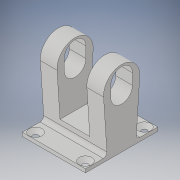
# Autodesk Inventor part: BT101_trajan20_21
Saved by Autodesk Inventor 2022.2 (Build 262287000, 287)
## iProperties
Company: HTBLA Kaindorf
RuleStatus: InUse
Created: 2022-08-03
Part Number: BT101_trajan20_21
Project: Zeichenmaschine_v2
Material: Generisch
Description: halterung
Document SubType Name: Modeling
Designer: trajan20
Density: 1 g/cm^3
Appearance: Vorgabe
Mass: 13.5366 g
Surface Area: 74.1019 cm^2
Volume: 13.5366 cm^3
AfterDocNew0: iProperties-Editor_aufrufen
Author: jan
Keywords: 2021
Autodesk Inventor part; units mm, degrees
ref_plane "YZ Plane" through (0, 0, 0) normal (1, 0, 0) x (0, 1, 0)
ref_plane "XZ Plane" through (0, 0, 0) normal (0, 1, 0) x (-1, 0, 0)
ref_plane "XY Plane" through (0, 0, 0) normal (0, 0, 1) x (1, 0, 0)
sketch "Skizze3" plane through (0, 0, 0) normal (0, 0, 1) x (1, 0, 0)
  line L0 (0, 0) -> (-40, 0)
  line L1 (-40, 0) -> (-40, 35)
  line L2 (-40, 35) -> (0, 35)
  line L3 (0, 35) -> (0, 0)
  point P0 (-3.7, 3.7)
  dimension "d4" = 35
  dimension "d5" = 40
  dimension "d6" = 3.7
  dimension "d7" = 3.7
  constraints: 8 end point, 2 parallel, 1 horizontal, 1 perpendicular
  measures "d4" distance between parallel lines of L2 L0
  measures "d5" distance between parallel lines of L1 L3
  measures "d6" distance from line of L3 point (-3.7, 3.7)
  measures "d7" distance from line of L0 point (-3.7, 3.7)
sketch "Skizze4" plane through (0, 0, 0) normal (0, 1, 0) x (-1, 0, 0)
  line L0 (0, 0) -> (40, 0) projected
  line L1 (20, 0) -> (20, 40)
  line L2 (20, 33) -> (20, 27) construction
  line L3 (26, 33) -> (26, 27)
  line L4 (14, 27) -> (14, 33)
  arc A0 (26, 33) -> (14, 33) centre (20, 33) ccw
  arc A1 (14, 27) -> (26, 27) centre (20, 27) ccw
  circle A2 centre (20, 30) radius 10
  line L5 (29.9773, 29.3273) -> (28, 0)
  line L6 (10.0227, 29.3273) -> (12, 0)
  dimension "d8" = 40
  dimension "d9" = 10
  dimension "d10" = 12
  dimension "d11" = 6
  dimension "d12" = 8
  dimension "d13" = 8
  constraints: 14 end point, 7 point on circle, 6 tangent, 4 point on line, 3 centre point, 2 midpoint, 1 coincident, 1 parallel, 1 vertical
  measures "d8" distance of L1.start L1.end
  measures "d9" distance of L1.end point (20, 30)
  measures "d10" distance between parallel lines of L4 L3
  measures "d11" distance of L2.start L2.end
  measures "d12" distance of L1.start L6.end
  measures "d13" distance of L1.start L5.end
extrude "Extrusion3" add sketch "Skizze4" along normal blind 35 contours L6 A2 L1 L0 | L1 A2 L5 L0 | A2 L1 A0 L4 A1 | L1 A1 L3 A0 A2
extrude "Extrusion4" add sketch "Skizze3" against normal blind 2
hole "Bohrung1" at (-3.7, 3.7, 0) direction (0, 0, -1) diameter 2.459 depth 8.8 countersink diameter 7 countersink angle 90 thread size "M3x0.5" class "6H" standard "ISO Metric profile"
sketch "Skizze5" plane through (0, 0, 0) normal (1, 0, 0) x (0, 0, -1)
  line L0 (-40, 0) -> (-40, 35) projected
  line L1 (-40, 9.25) -> (-5, 9.25)
  line L2 (-5, 9.25) -> (-5, 25.75)
  line L3 (-5, 25.75) -> (-40, 25.75)
  line L4 (-40, 25.75) -> (-40, 9.25)
  point P0 (0, 0)
  point P1 (-40, 17.5)
  dimension "d25" = 16.5
  dimension "d26" = 35
  constraints: 8 end point, 2 midpoint, 2 parallel, 1 horizontal, 1 perpendicular, 1 point on line
  measures "d25" distance between parallel lines of L3 L1
  measures "d26" distance between parallel lines of L0 L2
extrude "Extrusion5" cut sketch "Skizze5" against normal through all
pattern_linear "Rechteckige Anordnung1" count 2 spacing 32.6 along (-1, 0, 0) count 2 spacing 27.6 along (0, 1, 0) of "Bohrung1"
fillet "Rundung2" radius 2 2 edges at (-12, 17.5, 0) (-28, 17.5, 0)
equation "\"d7\" = d6"
equation "\"d13\" = d12"
equation "\"d14\" = d4"
equation "\"d31\" = d5 - 2 * d6"
equation "\"d34\" = d4 - 2 * d7"
